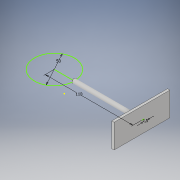
# Autodesk Inventor part: Kreisverkehrsschild_Teil_Unten
Saved by Autodesk Inventor 2019.5 (Build 235369000, 369)
## iProperties
Created: 2021-09-30
Part Number: Kreisverkehrsschild_Teil_Unten
Material: Generisch
Document SubType Name: Modeling
Designer: mritt
Density: 1 g/cm^3
Appearance: Vorgabe
Author: mritt
Autodesk Inventor part; units mm, degrees
ref_plane "YZ Plane" through (0, 0, 0) normal (1, 0, 0) x (0, 1, 0)
ref_plane "XZ Plane" through (0, 0, 0) normal (0, 1, 0) x (-1, 0, 0)
ref_plane "XY Plane" through (0, 0, 0) normal (0, 0, 1) x (1, 0, 0)
sketch "Skizze1" plane through (0, 0, 0) normal (0, 1, 0) x (-1, 0, 0)
  circle A0 centre (32.7504, -19.9257) radius 25
  line L0 (32.7504, -19.9257) -> (-77.2496, -19.9257)
  line L1 (-77.2496, -19.9257) -> (-77.2496, -22.4257)
  line L2 (-77.2496, -22.4257) -> (7.8757, -22.4257)
  line L3 (7.8757, -22.4257) -> (7.8757, -19.9257)
  point P0 (0, 0)
  dimension "d4" = 50
  dimension "d9" = 110
  dimension "d10" = 2.5
  constraints: 8 end point, 2 horizontal, 1 perpendicular, 1 point on line, 1 vertical, 3 other
  measures "d9" distance of L0.start L0.end
  measures "d10" distance of L0.end L1.end
extrude "Extrusion1" add sketch "Skizze1" along normal blind 1.5 and the other way blind 1.5 contours L3 L0 A0 | A0 L0 L3
revolve "Umdrehung1" add sketch "Skizze1" angle 360 about axis through (-32.7504, 0, -19.9257) along (1, 0, 0) picked at (7.8525, -21.3151) contours L2 L1 L0 A0 | A0 L0 L3
sketch "Skizze2" plane through (77.2496, 0, -19.9257) normal (1, 0, 0) x (0, 0, -1)
  line L0 (35, -15) -> (-35, -15)
  line L1 (-35, -15) -> (-35, 15)
  line L2 (-35, 15) -> (35, 15)
  line L3 (35, 15) -> (35, -15)
  line L4 (-25, -1.5) -> (25, 1.5)
  line L5 (35, -15) -> (-35, 15) construction
  line L6 (-35, -15) -> (35, 15) construction
  circle A0 centre (0, 0) radius 2.5 projected
  point P0 (-19.9257, 0)
  point P1 (0, 0)
  point P2 (-3.75, 0)
  point P3 (3.75, 0)
  point P4 (-25, -1.5)
  point P5 (25, 1.5)
  dimension "d14" = 70
  dimension "d15" = 30
  dimension "d22" = 15
  constraints: 12 end point, 2 midpoint, 2 parallel, 1 horizontal, 1 perpendicular, 4 other
  measures "d14" distance of L1.end L2.end
  measures "d15" distance of L0.end L1.end
  measures "d22" distance from line of A0.centre L2
extrude "Extrusion2" add sketch "Skizze2" against normal blind 3 contours L0 L1 L2 L3 | A0 L4 | L4 A0
sketch "Skizze3" plane through (0, 1.5, 0) normal (0, 1, 0) x (1, 0, 0)
  line L0 (-7.8305, 17.9257) -> (-7.8757, 17.9257) projected
  line L1 (-7.8757, 17.9257) -> (-59.898, 17.9257)
  line L2 (-59.898, 17.9257) -> (-59.898, 68.635)
  line L3 (-59.898, 68.635) -> (-7.8757, 68.635)
  line L4 (-7.8757, 68.635) -> (-7.8757, 17.9257)
  line L5 (-7.8757, 17.9257) -> (-59.898, 17.9257)
  line L6 (-59.898, 17.9257) -> (-59.898, -26.6959)
  line L7 (-59.898, -26.6959) -> (-7.8757, -26.6959)
  line L8 (-7.8757, -26.6959) -> (-7.8757, 17.9257)
  point P0 (0, 0)
  constraints: 16 end point, 4 parallel, 2 horizontal, 2 perpendicular, 1 point on line
extrude "Extrusion3" cut sketch "Skizze3" against normal blind 10
